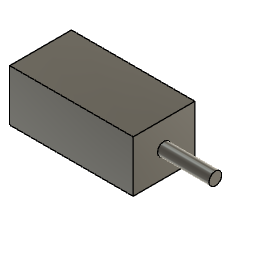
Moteur v2 (Autodesk Fusion 360 design; units mm, degrees)
Autodesk Fusion 360 part; units mm, degrees
sketch "Esquisse1" plane through (0, 0, 0) normal (0, 0, 1) x (1, 0, 0)
  line L0 (0, 0) -> (2.4, 0)
  line L1 (2.4, 0) -> (2.4, 1.2)
  line L2 (2.4, 1.2) -> (0, 1.2)
  line L3 (0, 1.2) -> (0, 0)
  dimension "d1" = 2.4
  dimension "d2" = 1.2
  constraint horizontal L0
  constraint vertical L1
  constraint horizontal L2
  constraint vertical L3
  constraint coincident L0.start L3.end
  measures "d1" distance of L0.start L0.end
  measures "d2" distance of L0.end L2
extrude "Extrusion1" add sketch "Esquisse1" along normal blind 1
sketch "Esquisse2" plane through (2.4, 0, 0) normal (1, 0, 0) x (0, 1, 0)
  line L0 (0, 0) -> (1.2, 0)
  line L1 (1.2, 0) -> (1.2, 1)
  line L2 (1.2, 1) -> (0, 1)
  line L3 (0, 1) -> (0, 0)
  circle A0 centre (0.6, 0.5) radius 0.125
  dimension "d5" = 0.25
  measures "d5" diameter of A0
extrude "Extrusion2" add sketch "Esquisse2" along normal blind 1 contours A0
scale "Echelle1" factor 10 about (0, 1.2, 1) bodies 1
